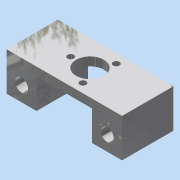
# Autodesk Inventor part: B Arm
Saved by Autodesk Inventor 2015 (Build 190159000, 159)
## iProperties
Created: 2017-11-13
Part Number: B Arm
Material: Generisch
Document SubType Name: Modeling
Designer: Christoph Soppa
Density: 1 g/cm^3
Appearance: Aluminium - poliert
Author: Christoph Soppa
Autodesk Inventor part; units mm, degrees
ref_plane "YZ Plane" through (0, 0, 0) normal (1, 0, 0) x (0, 1, 0)
ref_plane "XZ Plane" through (0, 0, 0) normal (0, 1, 0) x (-1, 0, 0)
ref_plane "XY Plane" through (0, 0, 0) normal (0, 0, 1) x (1, 0, 0)
sketch "Skizze1" plane through (0, 0, 0) normal (0, 0, 1) x (1, 0, 0)
  circle A0 centre (0, 0) radius 6.5
  line L0 (-27, 12) -> (27, 12)
  line L1 (27, 12) -> (27, -12)
  line L2 (27, -12) -> (-27, -12)
  line L3 (-27, -12) -> (-27, 12)
  dimension "d0" = 13
  dimension "d1" = 24
  dimension "d2" = 12
  dimension "d3" = 54
  dimension "d4" = 27
  constraints: 8 end point, 2 parallel, 1 centre point, 1 coincident, 1 horizontal, 1 perpendicular
  measures "d0" diameter of A0
  measures "d1" distance of L0.end L1.end
  measures "d2" distance from line of L0 point (0, 0)
  measures "d3" distance of L0.start L0.end
  measures "d4" distance from line of L1 point (0, 0)
extrude "Extrusion1" add sketch "Skizze1" along normal blind 4
sketch "Skizze2" plane through (0, 0, 0) normal (0, 0, -1) x (-1, 0, 0)
  line L0 (-27, -12) -> (-13, -12)
  line L1 (-13, -12) -> (-13, 12)
  line L2 (-13, 12) -> (-27, 12)
  line L3 (-27, 12) -> (-27, -12)
  line L4 (13, -12) -> (27, -12)
  line L5 (27, -12) -> (27, 12)
  line L6 (27, 12) -> (13, 12)
  line L7 (13, 12) -> (13, -12)
  point P0 (0, 0)
  dimension "d7" = 14
  dimension "d8" = 14
  dimension "d9" = 24
  dimension "d10" = 24
  dimension "d11" = 27
  dimension "d12" = 27
  dimension "d13" = 12
  constraints: 16 end point, 4 parallel, 2 horizontal, 2 perpendicular, 1 point on line
  measures "d7" distance of L1.end L2.end
  measures "d8" distance of L5.end L6.end
  measures "d9" distance of L0.end L1.end
  measures "d10" distance of L6.end L4.start
  measures "d11" distance from line of point (0, 0) L3
  measures "d12" distance from line of point (0, 0) L5
  measures "d13" distance from line of L2 point (0, 0)
extrude "Extrusion2" add sketch "Skizze2" along normal blind 14
hole "Bohrung1" at (20, 12, -7) direction (0, -1, 0) diameter 6.1 depth 24
hole "Bohrung2" at (-20, 12, -7) direction (0, -1, 0) diameter 6.1 depth 724
hole "Bohrung3" at (-9, 0, 4) direction (0, 0, -1) diameter 3 depth 8 tip angle 118
pattern_circular "Runde Anordnung1" count 3 over 360 about axis through (0, 0, 0) along (0, 0, 1) of "Bohrung3"
